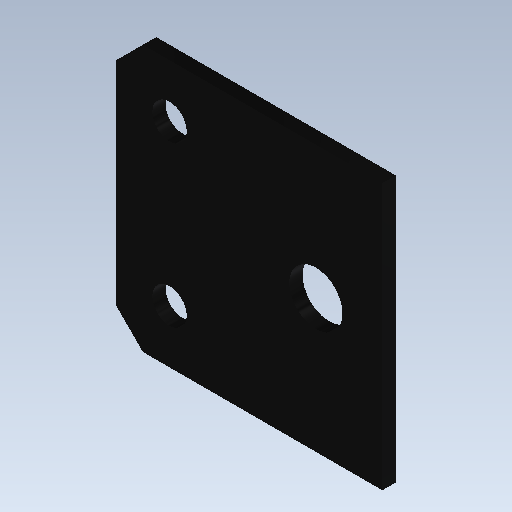
# Autodesk Inventor part: ADSK-MH-10042
Saved by Autodesk Inventor 2020.2 (Build 242310000, 310)
## iProperties
Created: 2008-03-10
Part Number: ADSK-MH-10042
Document SubType Name: Modeling
Designer: R.O'mahony
Density: 7.86 g/cm^3
Mass: 366.291 g
Surface Area: 213.047 cm^2
Volume: 46.6019 cm^3
Material: Steel, Mild
Description: Foot Plate
Appearance: Glossy - Black
Engineer: Demir Ali
Checked By: Demir Ali
Company: Autodesk Ltd
Author: R.O'mahony
Keywords: Roller Conveyor
Revision Number: A
Autodesk Inventor part; units mm, degrees
ref_plane "YZ Plane" through (0, 0, 0) normal (1, 0, 0) x (0, 1, 0)
ref_plane "XZ Plane" through (0, 0, 0) normal (0, 1, 0) x (-1, 0, 0)
ref_plane "XY Plane" through (0, 0, 0) normal (0, 0, 1) x (1, 0, 0)
sketch "Sketch1" plane through (0, 0, 0) normal (0, 0, 1) x (1, 0, 0)
  line L0 (2537.2814, -518.9919) -> (2551.2814, -527.0748)
  line L1 (2551.2814, -527.0748) -> (2565.2814, -518.9919)
  line L2 (2565.2814, -518.9919) -> (2565.2814, -502.826)
  line L3 (2565.2814, -502.826) -> (2551.2814, -494.7431)
  line L4 (2551.2814, -494.7431) -> (2537.2814, -502.826)
  line L5 (2537.2814, -502.826) -> (2537.2814, -518.9919)
  line L6 (2476.2814, -470.9089) -> (2476.2814, -550.9089)
  line L7 (2476.2814, -550.9089) -> (2486.2814, -560.9089)
  line L8 (2486.2814, -560.9089) -> (2576.2814, -560.9089)
  line L9 (2576.2814, -560.9089) -> (2576.2814, -460.9089)
  line L10 (2576.2814, -460.9089) -> (2486.2814, -460.9089)
  line L11 (2486.2814, -460.9089) -> (2476.2814, -470.9089)
  circle A0 centre (2496.2814, -540.9089) radius 6.5
  circle A1 centre (2496.2814, -480.9089) radius 6.5
  circle A2 centre (2551.2814, -510.9089) radius 10
  point P0 (0, 0)
  dimension "d1" = 80
  dimension "d3" = 25
  dimension "d5" = 100
  dimension "d7" = 13
  dimension "d9" = 100
  dimension "d11" = 50
  dimension "d13" = 20
  dimension "d15" = 20
  constraints: 24 end point, 3 centre point
  measures "d1" horizontal distance of L9.end A1.centre
  measures "d3" distance from line of A2.centre L9
  measures "d5" horizontal distance of L9.end L6.start
  measures "d7" diameter of A1
  measures "d9" distance of L9.end L8.end
  measures "d11" vertical distance of L9.end A2.centre
  measures "d13" vertical distance of L10.end A1.centre
  measures "d15" vertical distance of L7.end A0.centre
extrude "Extrusion1" add sketch "Sketch1" along normal blind 5 contours L5 L4 L3 L2 L1 L0 | L11 L10 L9 L8 L7 L6
body "Solid1"
